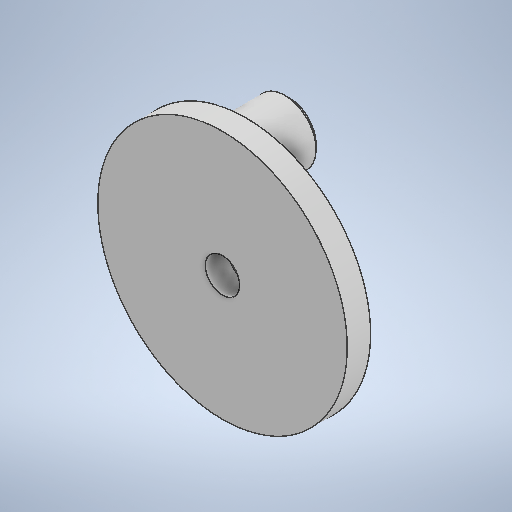
# Autodesk Inventor part: adapter_xl320
Saved by Autodesk Inventor 2025 (Build 290162000, 162)
## iProperties
Created: 2025-10-23
Part Number: adapter_xl320
Material: 一般
Document SubType Name: Modeling
Designer: sooo1
Density: 1 g/cm^3
Appearance: 既定
Author: sooo1
Autodesk Inventor part; units mm, degrees
ref_plane "YZ Plane" through (0, 0, 0) normal (1, 0, 0) x (0, 1, 0)
ref_plane "XZ Plane" through (0, 0, 0) normal (0, 1, 0) x (-1, 0, 0)
ref_plane "XY Plane" through (0, 0, 0) normal (0, 0, 1) x (1, 0, 0)
sketch "スケッチ1" plane through (0, 0, 0) normal (0, 0, 1) x (1, 0, 0)
  circle A0 centre (0, 0) radius 8
  line L0 (-11.2, 0) -> (11.2, 0) construction
  line L1 (0, -11.2) -> (0, 11.2) construction
  circle A1 centre (0, 6) radius 2
  circle A2 centre (0, -6) radius 2
  circle A3 centre (0, 0) radius 1.1
  dimension "d0" = 16
  dimension "d1" = 4
  dimension "d2" = 6
  dimension "d10" = 2.2
  constraints: 4 centre point, 2 coincident, 1 point on line, 1 symmetric about line, 1 other
  measures "d0" diameter of A0
  measures "d1" diameter of A1
  measures "d2" distance from line of L0 A1.centre
  measures "d10" diameter of A3
extrude "押し出し1" add sketch "スケッチ1" along normal blind 1.5 contours A1 | A2 | A0 | A3
extrude "押し出し2" add sketch "スケッチ1" against normal blind 2.8 contours A1 | A2
chamfer "面取り1" distance 0.3 angle 45 2 edges at (-2, 6, -2.8) (-2, -6, -2.8)
extrude "押し出し3" cut sketch "スケッチ1" along normal blind 10 contours A3
